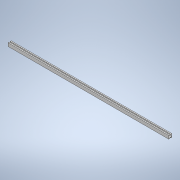
# Autodesk Inventor part: launchrail
Saved by Autodesk Inventor 2022 (Build 260153000, 153)
## iProperties
Created: 2021-05-16
Part Number: launchrail
Material: Generic
Document SubType Name: Modeling
Designer: shrec
Mass: 2354.32 g
Surface Area: 4496.41 cm^2
Volume: 2354.32 cm^3
Density: 1 g/cm^3
Appearance: Default
Author: shrec
Autodesk Inventor part; units mm, degrees
ref_plane "YZ Plane" through (0, 0, 0) normal (1, 0, 0) x (0, 1, 0)
ref_plane "XZ Plane" through (0, 0, 0) normal (0, 1, 0) x (-1, 0, 0)
ref_plane "XY Plane" through (0, 0, 0) normal (0, 0, 1) x (1, 0, 0)
sketch "Sketch1" plane through (0, 0, 0) normal (1, 0, 0) x (0, 1, 0)
  line L0 (20, 20) -> (-20, 20)
  arc A0 (5.6, -19.2) -> (-5.6, -19.2) centre (0, -15) ccw
  line L1 (-20, 20) -> (20, 20)
  arc A1 (19.2, 5.6) -> (19.2, -5.6) centre (15, 0) ccw
  line L2 (-20, 20) -> (20, 20)
  arc A2 (-19.2, -5.6) -> (-19.2, 5.6) centre (-15, 0) ccw
  line L3 (20, 20) -> (-20, 20)
  line L4 (-20, -20) -> (-6, -20)
  line L5 (6, -20) -> (20, -20)
  line L6 (-20, 20) -> (-20, 6)
  line L7 (-20, -6) -> (-20, -20)
  line L8 (20, -20) -> (20, -6)
  line L9 (20, 6) -> (20, 20)
  line L10 (20, 20) -> (20, 6)
  line L11 (20, -6) -> (20, -20)
  line L12 (-20, -20) -> (-20, -6)
  line L13 (-20, 6) -> (-20, 20)
  arc A3 (19.2, 5.6) -> (20, 6) centre (19.5, 6) ccw
  arc A4 (20, -6) -> (19.2, -5.6) centre (19.5, -6) ccw
  arc A5 (-6, -20) -> (-5.6, -19.2) centre (-6, -19.5) ccw
  arc A6 (5.6, -19.2) -> (6, -20) centre (6, -19.5) ccw
  arc A7 (-19.2, -5.6) -> (-20, -6) centre (-19.5, -6) ccw
  arc A8 (-20, 6) -> (-19.2, 5.6) centre (-19.5, 6) ccw
  point P0 (0, 0)
  point P1 (-4.899, -20)
  point P2 (4.899, -20)
  dimension "d3" = 40
  dimension "d4" = 40
  dimension "d5" = 40
  dimension "d9" = 14
  dimension "d10" = 0.5
  dimension "d11" = 0.5
  constraints: 28 end point, 20 point on circle, 12 tangent, 9 centre point, 4 equal radius, 2 perpendicular, 2 point on line
  measures "d3" distance of L5.end L0.start
  measures "d4" distance of L0.start L0.end
  measures "d5" distance of L0.end L4.start
  measures "d9" diameter of A0
  measures "d10" radius of A3
  measures "d11" radius of A5
extrude "Extrusion1" add sketch "Sketch1" along normal mid plane 2000
body "Solid1"
